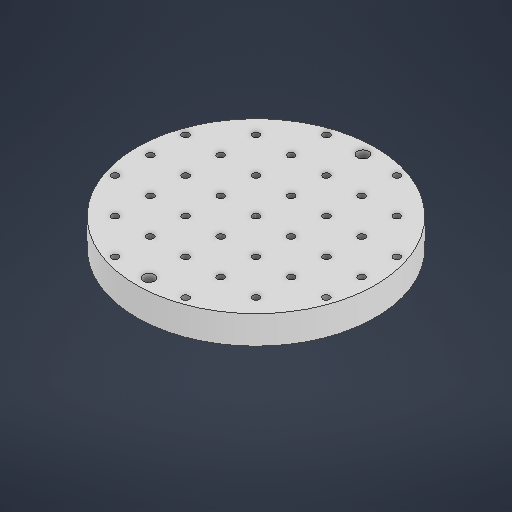
# Autodesk Inventor part: substrate plate With Lots of holes
Saved by Autodesk Inventor 2025 (Build 290162000, 162)
## iProperties
Created: 2024-06-21
Part Number: substrate plate With Lots of holes
Material: Generic
Document SubType Name: Modeling
Designer: mayhe
Density: 1 g/cm^3
Appearance: Default
Author: mayhe
Autodesk Inventor part; units mm, degrees
ref_plane "YZ Plane" through (0, 0, 0) normal (1, 0, 0) x (0, 1, 0)
ref_plane "XZ Plane" through (0, 0, 0) normal (0, 1, 0) x (-1, 0, 0)
ref_plane "XY Plane" through (0, 0, 0) normal (0, 0, 1) x (1, 0, 0)
sketch "Sketch1" plane through (0, 0, 0) normal (0, 1, 0) x (-1, 0, 0)
  circle A0 centre (0, 0) radius 84.75
  dimension "d0" = 169.5
  constraints: 1 centre point, 1 coincident
  measures "d0" diameter of A0
extrude "Extrusion1" add sketch "Sketch1" along normal blind 20
sketch "Sketch2" plane through (0, 0, 0) normal (0, -1, 0) x (1, 0, 0)
  circle A0 centre (0, 0) radius 76
  circle A1 centre (0, 76) radius 4
  circle A2 centre (0, -76) radius 4
  circle A3 centre (0, 76) radius 2.25
  circle A4 centre (0, -76) radius 2.25
  dimension "d3" = 152
  dimension "d4" = 8
  dimension "d5" = 8
  dimension "d6" = 4.5
  dimension "d7" = 4.5
  constraints: 5 centre point, 3 point on circle, 2 coincident
  measures "d3" diameter of A0
  measures "d4" diameter of A1
  measures "d5" diameter of A2
  measures "d6" diameter of A3
  measures "d7" diameter of A4
extrude "Extrusion2" cut sketch "Sketch2" against normal through all contours A3 A0 | A0 A3 | A4 A0 | A0 A4
extrude "Extrusion3" cut sketch "Sketch2" against normal blind 12 contours A1 A0 A3 | A0 A3 A1 | A2 A0 A4 | A0 A4 A2 | A3 A0 | A0 A3 | A4 A0 | A0 A4
sketch "Sketch3" plane through (0, 0, 0) normal (0, -1, 0) x (1, 0, 0)
  circle A0 centre (0, 0) radius 84.75 projected
  line L0 (59.9273, -59.9273) -> (59.9273, 59.9273)
  line L1 (59.9273, 59.9273) -> (-59.9273, 59.9273)
  line L2 (-59.9273, 59.9273) -> (-59.9273, -59.9273)
  line L3 (-59.9273, -59.9273) -> (59.9273, -59.9273)
  circle A1 centre (0, 0) radius 3
  circle A2 centre (-25, 0) radius 3
  circle A3 centre (-50, 0) radius 3
  circle A4 centre (0, 25) radius 3
  circle A5 centre (-25, 25) radius 3
  circle A6 centre (-50, 25) radius 3
  circle A7 centre (0, 50) radius 3
  circle A8 centre (-25, 50) radius 3
  circle A9 centre (-50, 50) radius 3
  line L4 (0, -59.9273) -> (0, 59.9273)
  line L5 (-59.9273, 0) -> (59.9273, 0)
  circle A10 centre (0, 0) radius 3
  circle A11 centre (25, 0) radius 3
  circle A12 centre (50, 0) radius 3
  circle A13 centre (0, 25) radius 3
  circle A14 centre (25, 25) radius 3
  circle A15 centre (50, 25) radius 3
  circle A16 centre (0, 50) radius 3
  circle A17 centre (25, 50) radius 3
  circle A18 centre (50, 50) radius 3
  circle A19 centre (0, 0) radius 3
  circle A20 centre (-25, 0) radius 3
  circle A21 centre (-50, 0) radius 3
  circle A22 centre (0, -50) radius 3
  circle A23 centre (50, 0) radius 3
  circle A24 centre (50, -25) radius 3
  circle A25 centre (50, -50) radius 3
  circle A26 centre (25, 0) radius 3
  circle A27 centre (25, -25) radius 3
  circle A28 centre (25, -50) radius 3
  circle A29 centre (0, 0) radius 3
  circle A30 centre (0, -25) radius 3
  circle A31 centre (0, -50) radius 3
  circle A32 centre (-25, 0) radius 3
  circle A33 centre (-50, 0) radius 3
  circle A34 centre (-25, -25) radius 3
  circle A35 centre (-50, -25) radius 3
  circle A36 centre (-25, -50) radius 3
  circle A37 centre (-50, -50) radius 3
  circle A38 centre (-25, 0) radius 3
  circle A39 centre (-50, 0) radius 3
  circle A40 centre (-75, -25) radius 3
  circle A41 centre (-50, 0) radius 3
  circle A42 centre (-75, 0) radius 3
  circle A43 centre (-50, 25) radius 3
  circle A44 centre (-75, 25) radius 3
  circle A45 centre (75, -25) radius 3
  circle A46 centre (75, 0) radius 3
  circle A47 centre (75, 25) radius 3
  circle A48 centre (0, -50) radius 3
  circle A49 centre (-25, -50) radius 3
  circle A50 centre (25, -75) radius 3
  circle A51 centre (0, -75) radius 3
  circle A52 centre (-25, -75) radius 3
  circle A53 centre (25, 75) radius 3
  circle A54 centre (-25, 75) radius 3
  dimension "d16" = 6
  dimension "d19" = 25
  dimension "d22" = 25
  dimension "d34" = 25
  dimension "d37" = 25
  dimension "d42" = 25
  dimension "d45" = 25
  constraints: 54 centre point, 22 symmetric about line, 12 end point, 4 midpoint, 4 vertical, 3 horizontal, 2 coincident, 2 parallel, 2 point on circle, 1 perpendicular, 71 other
  measures "d16" diameter of A1
  measures "d19" distance of A1.centre A2.centre
  measures "d22" distance of A1.centre A4.centre
  measures "d34" distance of A35.centre A40.centre
  measures "d37" distance of A35.centre A41.centre
  measures "d42" distance of A28.centre A48.centre
  measures "d45" distance of A28.centre A50.centre
hole "Hole1" at (-50, 0, -50) at (-50, 0, -25) at (-25, 0, -50) at (0, 0, -50) at (25, 0, -50) at (50, 0, -50) at (50, 0, -25) at (25, 0, -25) at (0, 0, -25) at (-25, 0, -25) at (-50, 0, 0) at (-25, 0, 0) at (0, 0, 0) at (25, 0, 0) at (50, 0, 0) at (50, 0, 25) at (25, 0, 25) at (0, 0, 25) at (-25, 0, 25) at (-50, 0, 25) at (-50, 0, 50) at (-25, 0, 50) at (0, 0, 50) at (25, 0, 50) at (50, 0, 50) at (25, 0, -75) at (-25, 0, -75) at (-25, 0, 75) at (25, 0, 75) at (75, 0, 25) at (75, 0, 0) at (75, 0, -25) at (-75, 0, -25) at (-75, 0, 0) at (-75, 0, 25) direction (0, 1, 0) diameter 4.917 depth 15 tip angle 118 thread size "M6x1" class "6H" standard "ANSI Metric M Profile"
body "Solid1"
